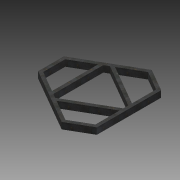
# Autodesk Inventor part: Platform
Saved by Autodesk Inventor 2015 SP1 (Build 190203100, 203)
## iProperties
Created: 2016-02-02
Part Number: Platform
Material: Steel
Document SubType Name: Modeling
Designer: tuttlem
Mass: 32237.8 g
Surface Area: 4761.07 cm^2
Volume: 4106.72 cm^3
Density: 7.85 g/cm^3
Appearance: Plate
Author: tuttlem
Autodesk Inventor part; units mm, degrees
ref_plane "YZ Plane" through (0, 0, 0) normal (1, 0, 0) x (0, 1, 0)
ref_plane "XZ Plane" through (0, 0, 0) normal (0, 1, 0) x (-1, 0, 0)
ref_plane "XY Plane" through (0, 0, 0) normal (0, 0, 1) x (1, 0, 0)
sketch "Sketch1" plane through (0, 0, 0) normal (0, 1, 0) x (-1, 0, 0)
  line L0 (613.6799, 122.9576) -> (173.739, 376.9576)
  line L1 (-2.2373, 275.3576) -> (-2.2373, -232.6424)
  line L2 (173.739, -334.2424) -> (613.6799, -80.2424)
  line L3 (613.6799, 122.9576) -> (613.6799, -80.2424)
  line L4 (173.739, 376.9576) -> (-2.2373, 275.3576)
  line L5 (173.739, -334.2424) -> (-2.2373, -232.6424)
  line L6 (588.2799, 108.2929) -> (173.739, 347.6282)
  line L7 (173.739, 347.6282) -> (23.1627, 260.6929)
  line L8 (23.1627, 260.6929) -> (23.1627, -217.9777)
  line L9 (23.1627, -217.9777) -> (173.739, -304.913)
  line L10 (173.739, -304.913) -> (588.2799, -65.5777)
  line L11 (588.2799, -65.5777) -> (588.2799, 108.2929)
  line L12 (397.9021, 218.2076) -> (397.9021, -175.4924)
  line L13 (364.1169, 237.7135) -> (23.1627, 40.8635)
  line L14 (364.1169, -194.9983) -> (23.1627, 1.8517)
  line L15 (338.7169, 252.3782) -> (23.1627, 70.1929)
  line L16 (23.1627, -27.4777) -> (338.7169, -209.663)
  line L17 (423.3021, 203.5429) -> (423.3021, -160.8277)
  point P0 (0, 0)
  dimension "d0" = 203.2
  dimension "d6" = 508
  dimension "d14" = 393.7
  dimension "d16" = 393.7
  dimension "d17" = 393.7
  constraints: 36 end point, 12 point on line, 8 parallel, 6 vertical, 6 other
  measures "d0" distance of L2.end L0.start
  measures "d6" distance of L0.end L0.start
  measures "d14" distance of L12.start L12.end
  measures "d16" distance of L13.start L13.end
  measures "d17" distance of L14.start L14.end
extrude "Extrusion1" add sketch "Sketch1" along normal blind 50.8 contours L3 L2 L5 L1 L4 L0 | L17 L10 L12 L6 | L13 L8 L15 L6 | L10 L16 L8 L14
body "Solid1"
